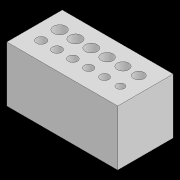
# Autodesk Inventor part: ThreadingTestBlock
Saved by Autodesk Inventor 2021 (Build 250183000, 183)
## iProperties
Created: 2021-01-21
Part Number: ThreadingTestBlock
Material: Generic
Document SubType Name: Modeling
Designer: Esketitttttt
Density: 1 g/cm^3
Appearance: Default
Author: Esketitttttt
Autodesk Inventor part; units mm, degrees
ref_plane "YZ Plane" through (0, 0, 0) normal (1, 0, 0) x (0, 1, 0)
ref_plane "XZ Plane" through (0, 0, 0) normal (0, 1, 0) x (-1, 0, 0)
ref_plane "XY Plane" through (0, 0, 0) normal (0, 0, 1) x (1, 0, 0)
sketch "Sketch1" plane through (0, 0, 0) normal (0, 1, 0) x (-1, 0, 0)
  line L0 (0, 0) -> (-25.4, 0)
  line L1 (-25.4, 0) -> (-25.4, -12.7)
  line L2 (-25.4, -12.7) -> (0, -12.7)
  line L3 (0, -12.7) -> (0, 0)
  line L4 (0, 0) -> (0, -4.2333)
  line L5 (0, 0) -> (0, -8.4667)
  line L6 (0, -4.2333) -> (-3.6286, -4.2333) construction
  line L7 (0, -8.4667) -> (-3.6286, -8.4667) construction
  circle A0 centre (-3.6286, -8.4667) radius 1.4224
  line L8 (-3.6286, -8.4667) -> (-7.2571, -8.4667) construction
  line L9 (-7.2571, -8.4667) -> (-10.8857, -8.4667) construction
  line L10 (-10.8857, -8.4667) -> (-14.5143, -8.4667) construction
  line L11 (-14.5143, -8.4667) -> (-18.1429, -8.4667) construction
  line L12 (-3.6286, -4.2333) -> (-7.2571, -4.2333) construction
  line L13 (-7.2571, -4.2333) -> (-10.8857, -4.2333) construction
  line L14 (-10.8857, -4.2333) -> (-14.5143, -4.2333) construction
  line L15 (-14.5143, -4.2333) -> (-18.1429, -4.2333) construction
  circle A1 centre (-3.6286, -4.2333) radius 1.0922
  line L16 (-18.1429, -4.2333) -> (-21.7714, -4.2333) construction
  line L17 (-21.7714, -4.2333) -> (-25.4, -4.2333) construction
  line L18 (-18.1429, -8.4667) -> (-21.7714, -8.4667) construction
  line L19 (-21.7714, -8.4667) -> (-25.4, -8.4667) construction
  circle A2 centre (-7.2571, -8.4667) radius 1.397
  circle A3 centre (-10.8857, -8.4667) radius 1.3716
  circle A4 centre (-14.5143, -8.4667) radius 1.3462
  circle A5 centre (-18.1429, -8.4667) radius 1.3208
  circle A6 centre (-21.7714, -8.4667) radius 1.2192
  circle A7 centre (-7.2571, -4.2333) radius 1.0668
  circle A8 centre (-10.8857, -4.2333) radius 1.0414
  circle A9 centre (-14.5143, -4.2333) radius 1.016
  circle A10 centre (-18.1429, -4.2333) radius 0.9906
  circle A11 centre (-21.7714, -4.2333) radius 0.889
  dimension "d0" = 25.4
  dimension "d1" = 12.7
  dimension "d2" = 4.2333
  dimension "d3" = 8.4667
  dimension "d4" = 3.6286
  dimension "d5" = 3.6286
  dimension "d6" = 2.8448
  dimension "d9" = 3.6286
  dimension "d14" = 3.6286
  dimension "d15" = 3.6286
  dimension "d16" = 3.6286
  dimension "d19" = 3.6286
  dimension "d24" = 3.6286
  dimension "d25" = 3.6286
  dimension "d26" = 3.6286
  dimension "d27" = 2.1844
  dimension "d28" = 2.794
  dimension "d29" = 2.7432
  dimension "d30" = 2.6924
  dimension "d31" = 3.6286
  dimension "d32" = 3.6286
  dimension "d33" = 3.6286
  dimension "d34" = 3.6286
  dimension "d35" = 3.6286
  dimension "d36" = 3.6286
  dimension "d37" = 2.6416
  dimension "d38" = 2.4384
  dimension "d39" = 2.1336
  dimension "d40" = 2.0828
  dimension "d41" = 2.032
  dimension "d42" = 1.9812
  dimension "d43" = 1.778
  constraints: 40 end point, 12 centre point, 12 coincident, 5 horizontal, 2 collinear, 2 parallel, 2 point on line, 1 perpendicular, 34 other
  measures "d0" distance of L2.end L1.end
  measures "d1" distance of L1.end L0.end
  measures "d2" distance of L0.start L4.end
  measures "d3" distance of L0.start L5.end
  measures "d4" distance of L4.end L6.end
  measures "d5" distance of L5.end L7.end
  measures "d6" diameter of A0
  measures "d9" distance of L5.end L8.start
  measures "d14" distance of L8.start L8.end
  measures "d15" distance of L9.start L9.end
  measures "d16" distance of L10.start L10.end
  measures "d19" distance of L4.end L12.start
  measures "d24" distance of L12.start L12.end
  measures "d25" distance of L13.start L13.end
  measures "d26" distance of L14.start L14.end
  measures "d27" diameter of A1
  measures "d28" diameter of A2
  measures "d29" diameter of A3
  measures "d30" diameter of A4
  measures "d31" distance of L11.start L11.end
  measures "d32" distance of L18.start L18.end
  measures "d33" distance of L19.start L19.end
  measures "d34" distance of L15.start L15.end
  measures "d35" distance of L16.start L16.end
  measures "d36" distance of L17.start L17.end
  measures "d37" diameter of A5
  measures "d38" diameter of A6
  measures "d39" diameter of A7
  measures "d40" diameter of A8
  measures "d41" diameter of A9
  measures "d42" diameter of A10
  measures "d43" diameter of A11
extrude "Extrusion1" add sketch "Sketch1" along normal blind 12.7
equation "\"d2\" = 0.333333 * d1"
equation "\"d3\" = 0.666667 * d1"
equation "\"d4\" = d5"
equation "\"d5\" = 0.142857 * d0"
equation "\"d9\" = d5"
equation "\"d19\" = d4"
body "Solid1"
